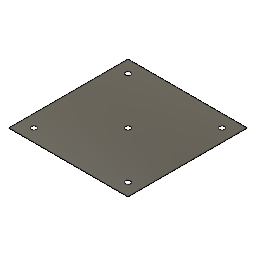
heater v6 (Autodesk Fusion 360 design; units mm, degrees)
Autodesk Fusion 360 part; units mm, degrees
sketch "Sketch2" plane through (0, 0, 0) normal (0, 0, 1) x (1, 0, 0)
  line L0 (152.5, -152.5) -> (-152.5, -152.5)
  line L1 (-152.5, -152.5) -> (-152.5, 152.5)
  line L2 (-152.5, 152.5) -> (152.5, 152.5)
  line L3 (152.5, 152.5) -> (152.5, -152.5)
  line L4 (120, -120) -> (-120, -120)
  line L5 (-120, -120) -> (-120, 120)
  line L6 (-120, 120) -> (120, 120)
  line L7 (120, 120) -> (120, -120)
  line L8 (120, -120) -> (-120, 120) construction
  line L9 (-120, -120) -> (120, 120) construction
  circle A0 centre (120, 120) radius 6
  circle A1 centre (-120, 120) radius 6
  circle A2 centre (-120, -120) radius 6
  circle A3 centre (120, -120) radius 6
  circle A4 centre (0, 0) radius 6
  dimension "d6" = 305
  dimension "d7" = 305
  dimension "d8" = 240
  dimension "d9" = 240
  dimension "d10" = 12
  dimension "d12" = 360
  dimension "d15" = 12
  constraint perpendicular L0 L1
  constraint parallel L0 L2
  constraint parallel L1 L3
  constraint horizontal L0
  constraint coincident A4.centre origin
  constraint perpendicular L4 L5
  constraint parallel L4 L6
  constraint parallel L5 L7
  constraint horizontal L4
  constraint coincident L8 A4.centre
  constraint coincident L9 A4.centre
  constraint coincident L6.end L7.start
  measures "d6" distance of L1.end L2.end
  measures "d7" distance of L0.end L1.end
  measures "d8" distance of L4.end L5.end
  measures "d9" distance of L5.end L6.end
  measures "d10" diameter of A0
  measures "d15" diameter of A4
extrude "Extrude1" add sketch "Sketch2" along normal blind 1 contours L0 L1 L2 L3 | L4 L5 L6 L7 A0 A1 A2 A3
